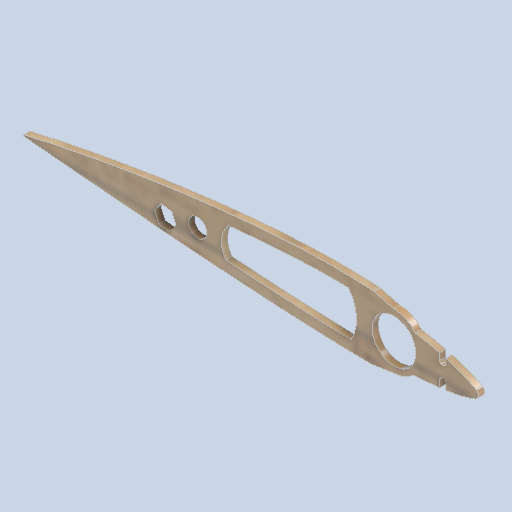
# Autodesk Inventor part: Rib V6 Flap BB
Saved by Autodesk Inventor 2025.2 (Build 292293000, 293)
## iProperties
Created: 2024-10-23
Part Number: Rib V6 Flap BB
Material: Wood (Maple)
Document SubType Name: Modeling
Designer: 17jo6
Density: 0.67 g/cm^3
Appearance: Natural Maple - Glossy Dark Tint
Author: 17jo6
Autodesk Inventor part; units mm, degrees
ref_plane "YZ Plane" through (0, 0, 0) normal (1, 0, 0) x (0, 1, 0)
ref_plane "XZ Plane" through (0, 0, 0) normal (0, 1, 0) x (-1, 0, 0)
ref_plane "XY Plane" through (0, 0, 0) normal (0, 0, 1) x (1, 0, 0)
sketch "Sketch1" plane through (0, 0, 0) normal (0, 0, 1) x (1, 0, 0)
  spline S0 degree 4 poles (254.436054, 38.258138) (252.159915, 38.650332) (246.788709, 39.499265) (237.984874, 40.618279) (225.357478, 41.704285) (211.202741, 42.341661) (196.392584, 42.47009) (181.031283, 42.070233) (165.506388, 41.221743) (149.785249, 40.04478) (134.1096, 38.577548) (118.624688, 36.850842) (103.500036, 34.939301) (88.901638, 32.883406) (74.995754, 30.738214) (61.917783, 28.562704) (49.827113, 26.40977) (38.835364, 24.340018) (29.07721, 22.403865) (20.632296, 20.65644) (13.645605, 19.149082) (6.913163, 17.660714) (2.90218, 16.740022) (0.469137, 16.188187) (0, 16.065) knots 0.21429705 0.21429705 0.21429705 0.21429705 0.21429705 0.2433201 0.28177524 0.32154178 0.36237973 0.40400459 0.44617789 0.48866482 0.5312306 0.57368816 0.61580317 0.65733642 0.6980466 0.73768213 0.77598623 0.81268845 0.84749504 0.88008735 0.91009265 0.93705903 0.9603631 1 1 1 1 1
  spline S1 degree 4 poles (299.999998, 15.624) (299.805651, 13.312974) (297.70854, 10.343184) (293.050897, 7.5008) (285.395888, 4.883043) (278.112378, 3.216454) (269.51472, 1.892454) (259.681019, 0.912997) (248.712883, 0.278332) (236.711867, -0.030891) (223.806667, -0.050368) (210.125319, 0.193333) (195.775416, 0.645033) (180.96771, 1.249367) (165.65166, 1.982539) (150.191633, 2.90484) (134.687258, 3.945111) (119.337536, 5.049498) (104.304232, 6.19869) (89.75661, 7.356132) (75.849241, 8.488651) (62.742943, 9.582403) (50.581067, 10.622604) (39.497088, 11.57965) (29.629376, 12.451281) (21.071247, 13.226368) (13.963939, 13.872105) (7.103576, 14.512622) (2.968279, 14.899676) (0.533018, 15.1397) (-0.004161, 15.184114) knots 0 0 0 0 0 0.05437224 0.07982113 0.10791215 0.1384988 0.1713415 0.2061871 0.24278378 0.28089063 0.3202767 0.36071301 0.4020228 0.44398485 0.4863729 0.52895769 0.5714601 0.61364209 0.65526508 0.6960853 0.73585299 0.77430798 0.81117416 0.84615676 0.87892978 0.90911464 0.93625212 0.9597112 1 1 1 1 1
  arc A0 (0, 16.065) -> (-0.004161, 15.184114) centre (0.115799, 15.624) ccw
  line L0 (0.115799, 15.624) -> (227.990221, 15.624) construction
  line L1 (299.999998, 15.624) -> (0.115799, 15.624) construction
  line L2 (299.999998, 15.624) -> (199.999998, 15.624) construction
  line L3 (199.999998, 15.624) -> (199.999998, 42.37734) construction
  line L4 (199.999998, 15.624) -> (199.999998, 0.52729)
  line L5 (0, 0) -> (0, 20.241)
  line L6 (0, 20.241) -> (238.581, 20.241) construction
  circle A1 centre (238.581, 20.241) radius 14
  line L7 (238.581, 20.241) -> (208.581, 20.241)
  line L8 (238.581, 25.359) -> (238.581, 20.241)
  line L9 (0, 20.241) -> (112, 20.241) construction
  circle A2 centre (112, 20.241) radius 5.39
  line L10 (0, 15.624) -> (112, 15.624) construction
  line L11 (0, 15.624) -> (112, 15.624) construction
  line L12 (112, 15.624) -> (112, 35.994456)
  line L13 (112, 15.624) -> (112, 5.61525)
  spline S2 degree 4 poles (299.285198, 20.241) (299.227939, 20.131643) (299.16804, 20.023225) (299.105573, 19.915754) (299.040612, 19.809235) knots 0 0 0 0 0 1 1 1 1 1
  line L14 (299.207055, 20.082158) -> (298.87417, 19.536312) construction
  arc A3 (298.903999, 19.593162) -> (299.170168, 20.029611) centre (292.291091, 23.925437) ccw construction
  line L15 (299.43203, 20.521431) -> (299.138367, 19.960569) construction
  arc A4 (299.163926, 20.01882) -> (299.398715, 20.467241) centre (292.801001, 23.636075) ccw construction
  spline S3 degree 2 poles (295.850621, 16.559978) (295.157262, 16.069203) (294.393311, 15.624) knots 0 0 0 1 1 1
  line L16 (294.550692, 15.715716) -> (294.235931, 15.532284) construction
  arc A5 (294.267154, 15.551069) -> (294.518956, 15.69781) centre (283.884356, 33.65696) ccw construction
  spline S4 degree 4 poles (296.856901, 15.624) (296.618326, 15.862944) (296.370731, 16.098547) (296.114674, 16.330852) (295.850621, 16.559978) knots 0 0 0 0 0 1 1 1 1 1
  spline S5 degree 4 poles (219.58717, 34.91187) (218.695351, 34.95198) (214.858509, 35.106335) (210.707211, 35.329502) (192.898023, 35.446366) (181.42777, 35.055508) (165.177387, 34.181901) (149.561876, 33.12667) (133.828431, 31.347909) (128.265438, 31.097419) (123.390775, 30.590026) knots 0 0 0 0 0 0.13924435 0.23321956 0.36393672 0.50998276 0.65711487 0.7981047 1 1 1 1 1
  line L17 (295.959293, 16.465681) -> (295.74195, 16.654276) construction
  arc A6 (295.937354, 16.484307) -> (295.763482, 16.635181) centre (281.87292, 0.451609) ccw construction
  line L18 (232.743774, 34.364452) -> (201.193566, 35.681454) construction
  arc A7 (229.586762, 34.454933) -> (204.347135, 35.508511) centre (136.348344, -1896.324468) ccw construction
  arc A8 (264.266057, 15.123) -> (264.360826, 15.624) centre (238.581, 20.241) ccw
  circle A9 centre (238.581, 20.241) radius 24
  circle A10 centre (112, 20.241) radius 15.39
  spline S6 degree 4 poles (299.999998, 15.624) (300.269142, 17.933652) (298.783415, 21.267693) (294.693448, 24.979847) (287.53174, 28.940551) (280.486947, 31.820538) (271.480983, 34.718213) (262.486804, 36.793013) (257.700386, 37.695672) (254.436054, 38.258138) knots 0 0 0 0 0 0.24755477 0.36385739 0.4925498 0.63299607 0.77826439 1 1 1 1 1
  line L19 (285.294543, 32.941011) -> (223.577565, 43.575266) construction
  arc A11 (278.722442, 32.634865) -> (229.668212, 41.087243) centre (217.218351, -177.738587) ccw construction
  line L20 (285.294543, 32.941011) -> (223.577565, 43.575266) construction
  arc A12 (278.877125, 33.041766) -> (229.658629, 41.522447) centre (200.894914, -272.473312) ccw construction
  spline S7 degree 4 poles (251.493, 31.73616) (243.700929, 32.967588) (232.160237, 34.296592) (216.442824, 35.287928) (196.392341, 35.461091) (181.031705, 35.061513) (165.505292, 34.212684) (149.788285, 33.036509) (134.101234, 31.567156) (118.647366, 29.846206) (103.439709, 27.919279) (89.058912, 25.903716) (74.837064, 23.692714) (62.488433, 21.669546) (49.639937, 19.354465) (46.379459, 18.742869) (43.812536, 18.259032) knots 0 0 0 0 0 0.1639631 0.23233838 0.3020312 0.37264227 0.44377843 0.51504665 0.58613365 0.65664712 0.72618654 0.7943479 0.86070997 0.92034602 1 1 1 1 1
  spline S8 degree 4 poles (295.845009, 16.556007) (295.719822, 16.664559) (294.584958, 17.628339) (292.058546, 19.428263) (287.516704, 21.93465) (280.467029, 24.832118) (271.97142, 27.522599) (264.208658, 29.400369) (258.409244, 30.551465) (255.053616, 31.142888) (254.436054, 31.249298) (253.968946, 31.329784) (253.501839, 31.41027) (253.034731, 31.490756) (252.567623, 31.571241) knots 0 0 0 0 0 0.01890503 0.16895946 0.33499927 0.51620401 0.71116085 0.9183366 0.96483207 0.96483207 0.96483207 0.96483207 1 1 1 1 1
  line L21 (285.294543, 25.932171) -> (223.577565, 36.566425) construction
  line L22 (285.294543, 25.932171) -> (223.577565, 36.566425) construction
  arc A13 (278.722442, 25.626025) -> (229.668212, 34.078402) centre (217.218351, -184.747428) ccw construction
  line L23 (270.129, 9.125374) -> (275.129, 9.125374) construction
  line L24 (281.07, 24.45816) -> (286.07, 24.45816) construction
  line L25 (318.821413, -3.367269) -> (272.868604, 36.479282) construction
  arc A14 (303.207925, 0.551953) -> (278.959518, 21.578206) centre (281.857648, 0.425162) ccw construction
  spline S9 degree 4 poles (295.835285, 16.564433) (293.417091, 14.88464) (288.41352, 12.692641) (280.70627, 10.669821) (269.511023, 8.939829) (259.682627, 7.96324) (248.712204, 7.32734) (236.712148, 7.018633) (223.806545, 6.998947) (210.125394, 7.242728) (195.775305, 7.694406) (180.967993, 8.298721) (165.65086, 9.03198) (150.193891, 9.954022) (134.681006, 10.995018) (119.354518, 12.097424) (104.258979, 13.251926) (89.874814, 14.39542) (75.752353, 15.547068) (62.906491, 16.616479) (50.510696, 17.677636) (46.516568, 18.024605) (43.812536, 18.259032) knots 0 0 0 0 0 0.08476672 0.12402522 0.16617938 0.21090431 0.25787677 0.30678758 0.35734028 0.40924097 0.46226281 0.51612182 0.5705276 0.62518592 0.67973848 0.7338798 0.78730362 0.83969707 0.89073959 0.93714265 1 1 1 1 1
  spline S10 degree 4 poles (21.462276, 20.241) (20.622656, 20.316984) (20.124028, 20.362207) (19.919133, 20.380856) (19.554048, 20.414029) knots 0 0 0 0 0 1 1 1 1 1 construction
  line L26 (68.488377, 16.119755) -> (19.136695, 20.398308) construction
  arc A15 (63.551474, 16.528056) -> (24.070206, 19.950891) centre (-819.899413, -9944.371227) ccw construction
  line L27 (21.724437, 20.217275) -> (21.200116, 20.264725) construction
  arc A16 (21.252548, 20.259982) -> (21.672005, 20.222022) centre (898.635849, 9712.955601) ccw construction
  line L28 (74.254065, 23.996937) -> (13.371006, 12.521126) construction
  arc A17 (68.175943, 22.793945) -> (19.469999, 13.613391) centre (1053.390082, -5337.891027) ccw construction
  spline S11 degree 4 poles (218.437499, 7.193419) (217.617295, 7.240848) (213.819214, 7.468804) (209.586315, 6.850678) (192.548492, 7.944114) (181.146901, 8.16297) (165.746092, 9.02826) (149.142366, 9.880106) (139.977668, 10.751942) (129.107316, 11.246393) (124.68665, 11.528881) knots 0 0 0 0 0 0.12763083 0.21372336 0.33362841 0.4674456 0.60262129 0.73842442 0.88039529 0.88039529 0.88039529 0.88039529 0.88039529
  line L29 (133.533683, 10.96354) -> (115.839617, 12.094223) construction
  arc A18 (117.617989, 12.078874) -> (131.767822, 11.174674) centre (141.026952, 267.238396) ccw construction
  line L30 (140.664975, 32.388062) -> (106.116576, 28.79199) construction
  arc A19 (137.221962, 31.449676) -> (109.679039, 28.58279) centre (140.622493, -134.959578) ccw construction
  circle A20 centre (238.581, 20.241) radius 18
  line L31 (238.581, 38.241) -> (225.78, 41.559)
  line L32 (238.581, 2.241) -> (224.22, 0)
  line L33 (214.581, 20.241) -> (214.581, 42.126574) construction
  line L34 (127.39, 20.241) -> (127.39, 11.525517) construction
  line L35 (127.39, 20.241) -> (131.31394, 20.241) construction
  line L36 (96.61, 20.241) -> (96.61, 13.863077) construction
  line L37 (270.129, 5.61525) -> (270.129, 15.624) construction
  line L38 (272.129, 7.61525) -> (272.129, 13.624)
  line L39 (268.129, 13.624) -> (268.129, 7.61525)
  arc A21 (268.129, 7.61525) -> (272.129, 7.61525) centre (270.129, 7.61525) ccw
  arc A22 (272.129, 13.624) -> (268.129, 13.624) centre (270.129, 13.624) ccw
  line L40 (270.129, 32.18075) -> (270.129, 22.172) construction
  line L41 (272.129, 30.18075) -> (272.129, 24.172)
  line L42 (268.129, 24.172) -> (268.129, 30.18075)
  arc A23 (272.129, 30.18075) -> (268.129, 30.18075) centre (270.129, 30.18075) ccw
  arc A24 (268.129, 24.172) -> (272.129, 24.172) centre (270.129, 24.172) ccw
  arc A25 (199.999998, 42.31547) -> (199.853854, 42.377258) centre (190.581, 20.241) ccw
  arc A26 (171.272979, 34.495835) -> (171.268099, 34.489223) centre (190.581, 20.241) ccw
  arc A27 (210.748391, 7.230376) -> (209.287499, 35.276521) centre (190.581, 20.241) ccw
  arc A28 (169.44554, 8.870309) -> (169.474435, 8.816763) centre (190.581, 20.241) ccw
  arc A29 (153.976817, 9.682431) -> (154.030254, 9.739387) centre (142.78, 20.241) ccw
  arc A30 (151.241916, 33.095886) -> (151.219343, 33.110716) centre (142.78, 20.241) ccw
  arc A31 (132.12991, 31.350801) -> (130.322928, 11.203663) centre (142.78, 20.241) ccw
  arc A32 (95.274104, 13.969298) -> (95.169771, 26.74146) centre (81.22, 20.241) ccw
  arc A33 (66.333989, 16.334751) -> (66.538876, 15.624) centre (81.22, 20.241) ccw
  line L43 (112, 20.241) -> (112, 14.851) construction
  circle A34 centre (91.265, 15.422) radius 4
  circle A35 centre (238.581, 20.241) radius 14.2
  circle A36 centre (112, 20.241) radius 5.92
  circle A37 centre (91.265, 15.422) radius 6
  line L44 (98.144895, 14.605275) -> (93.997643, 9.055474)
  line L45 (93.997643, 9.055474) -> (87.117748, 9.872198)
  line L46 (87.117748, 9.872198) -> (84.385105, 16.238725)
  line L47 (84.385105, 16.238725) -> (88.532357, 21.788526)
  line L48 (88.532357, 21.788526) -> (95.412252, 20.971802)
  line L49 (95.412252, 20.971802) -> (98.144895, 14.605275)
  point P0 (0.783, 16.254)
  point P1 (3.213, 16.812)
  point P2 (7.239, 17.724)
  point P3 (12.813, 18.96)
  point P4 (19.884, 20.484)
  point P5 (28.374, 22.245)
  point P6 (38.199, 24.195)
  point P7 (49.254, 26.28)
  point P8 (61.419, 28.446)
  point P9 (74.571, 30.636)
  point P10 (88.56, 32.793)
  point P11 (103.242, 34.86)
  point P12 (118.455, 36.783)
  point P13 (134.028, 38.511)
  point P14 (149.793, 39.984)
  point P15 (165.576, 41.16)
  point P16 (181.206, 41.985)
  point P17 (196.638, 42.363)
  point P18 (211.554, 42.222)
  point P19 (239.145, 40.389)
  point P20 (262.68, 36.666)
  point P21 (272.577, 34.218)
  point P22 (281.07, 31.467)
  point P23 (288.069, 28.491)
  point P24 (293.505, 25.359)
  point P25 (297.324, 22.137)
  point P26 (300, 15.624)
  point P27 (0.861, 15.105)
  point P28 (3.342, 14.868)
  point P29 (7.446, 14.481)
  point P30 (13.122, 13.953)
  point P31 (20.31, 13.296)
  point P32 (28.92, 12.519)
  point P33 (38.856, 11.64)
  point P34 (50.007, 10.674)
  point P35 (62.244, 9.63)
  point P36 (75.429, 8.529)
  point P37 (89.418, 7.389)
  point P38 (104.052, 6.228)
  point P39 (119.172, 5.076)
  point P40 (134.613, 3.966)
  point P41 (150.207, 2.928)
  point P42 (165.783, 2.013)
  point P43 (181.167, 1.263)
  point P44 (196.068, 0.663)
  point P45 (210.468, 0.225)
  point P46 (237.189, 0.039)
  point P47 (249.246, 0.378)
  point P48 (260.262, 1.05)
  point P49 (270.129, 2.076)
  point P50 (278.739, 3.462)
  point P51 (285.993, 5.211)
  point P52 (291.81, 7.314)
  point P53 (296.121, 9.756)
  point P54 (298.863, 12.531)
  point P55 (199.999998, 15.624)
  point P56 (225.364219, 15.624)
  point P57 (238.581, 6.241)
  point P58 (238.581, 34.241)
  point P59 (225.364219, 15.624)
  point P60 (251.797781, 15.624)
  point P61 (0, 16.065)
  point P62 (0, 15.183769)
  point P63 (224.581, 20.241)
  point P64 (112, 25.631)
  point P65 (0, 9.065)
  point P66 (0.783, 9.254)
  point P67 (3.213, 9.812)
  point P68 (7.239, 10.724)
  point P69 (12.813, 11.96)
  point P70 (19.884, 13.484)
  point P71 (28.374, 15.245)
  point P72 (38.199, 17.195)
  point P73 (49.254, 19.28)
  point P74 (61.419, 21.446)
  point P75 (74.571, 23.636)
  point P76 (88.56, 25.793)
  point P77 (103.242, 27.86)
  point P78 (118.455, 29.783)
  point P79 (134.028, 31.511)
  point P80 (149.793, 32.984)
  point P81 (165.576, 34.16)
  point P82 (181.206, 34.985)
  point P83 (225.78, 34.559)
  point P84 (239.145, 33.389)
  point P85 (251.493, 31.745)
  point P86 (262.68, 29.666)
  point P87 (272.577, 27.218)
  point P88 (281.07, 24.467)
  point P89 (288.069, 21.491)
  point P90 (293.505, 18.359)
  point P91 (297.324, 15.137)
  point P92 (299.493, 11.879)
  point P93 (300, 8.624)
  point P94 (-0.004161, 22.184114)
  point P95 (0.861, 22.105)
  point P96 (3.342, 21.868)
  point P97 (7.446, 21.481)
  point P98 (13.122, 20.953)
  point P99 (20.31, 20.296)
  point P100 (28.92, 19.519)
  point P101 (38.856, 18.64)
  point P102 (50.007, 17.674)
  point P103 (62.244, 16.63)
  point P104 (75.429, 15.529)
  point P105 (89.418, 14.389)
  point P106 (104.052, 13.228)
  point P107 (119.172, 12.076)
  point P108 (134.613, 10.966)
  point P109 (150.207, 9.928)
  point P110 (165.783, 9.013)
  point P111 (181.167, 8.263)
  point P112 (196.068, 7.663)
  point P113 (210.468, 7.225)
  point P114 (224.22, 7)
  point P115 (237.189, 7.039)
  point P116 (249.246, 7.378)
  point P117 (260.262, 8.05)
  point P118 (270.129, 9.076)
  point P119 (278.739, 10.462)
  point P120 (285.993, 12.211)
  point P121 (291.81, 14.314)
  point P122 (296.121, 16.756)
  point P123 (298.863, 19.531)
  point P124 (300, 22.624)
  point P125 (18.740477, 20.241)
  point P126 (216.96867, 35.022953)
  point P127 (0, 16.065)
  point P128 (296.856901, 15.624)
  point P129 (294.393311, 15.624)
  point P130 (219.58717, 34.91187)
  point P131 (123.390775, 30.590026)
  point P132 (254.436054, 38.258138)
  point P133 (0, 9.05616)
  point P134 (0.783, 9.24516)
  point P135 (3.213, 9.80316)
  point P136 (7.239, 10.71516)
  point P137 (12.813, 11.95116)
  point P138 (19.884, 13.47516)
  point P139 (28.374, 15.23616)
  point P140 (38.199, 17.18616)
  point P141 (49.254, 19.27116)
  point P142 (61.419, 21.43716)
  point P143 (74.571, 23.62716)
  point P144 (88.56, 25.78416)
  point P145 (103.242, 27.85116)
  point P146 (118.455, 29.77416)
  point P147 (134.028, 31.50216)
  point P148 (149.793, 32.97516)
  point P149 (165.576, 34.15116)
  point P150 (181.206, 34.97616)
  point P151 (196.638, 35.35416)
  point P152 (211.554, 35.21316)
  point P153 (225.78, 34.55016)
  point P154 (262.68, 29.65716)
  point P155 (272.577, 27.20916)
  point P156 (297.324, 15.12816)
  point P157 (299.493, 11.87016)
  point P158 (300, 8.61516)
  point P159 (254.436054, 31.249298)
  point P160 (216.884838, -206.362485)
  point P161 (278.876889, 26.073396)
  point P162 (229.590604, 33.866167)
  point P163 (-0.004161, 22.233488)
  point P164 (0.861, 22.154374)
  point P165 (3.342, 21.917374)
  point P166 (7.446, 21.530374)
  point P167 (13.122, 21.002374)
  point P168 (28.92, 19.568374)
  point P169 (38.856, 18.689374)
  point P170 (50.007, 17.723374)
  point P171 (62.244, 16.679374)
  point P172 (75.429, 15.578374)
  point P173 (89.418, 14.438374)
  point P174 (104.052, 13.277374)
  point P175 (119.172, 12.125374)
  point P176 (134.613, 11.015374)
  point P177 (150.207, 9.977374)
  point P178 (165.783, 9.062374)
  point P179 (181.167, 8.312374)
  point P180 (196.068, 7.712374)
  point P181 (210.468, 7.274374)
  point P182 (224.22, 7.049374)
  point P183 (237.189, 7.088374)
  point P184 (249.246, 7.427374)
  point P185 (260.262, 8.099374)
  point P186 (278.739, 10.511374)
  point P187 (285.993, 12.260374)
  point P188 (296.121, 16.805374)
  point P189 (298.863, 19.580374)
  point P190 (300, 22.673374)
  point P191 (225.700031, -0.009448)
  point P192 (252.261653, 0.521981)
  point P193 (227.349521, 41.450759)
  point P194 (105.977751, 6.07821)
  point P195 (115.800844, 5.327728)
  point P196 (98.259993, 27.173842)
  point P197 (260.452219, 30.122789)
  point P198 (123.585295, 30.371797)
  point P199 (134.59788, 31.560388)
  dimension "d38" = 10.78
  dimension "d68" = 12
  dimension "d17" = 100
  dimension "d19" = 20.241
  dimension "d20" = 238.581
  dimension "d21" = 28
  dimension "d37" = 112
  dimension "d39" = 112
  dimension "d40" = 0
  dimension "d43" = 10
  dimension "d44" = 10
  dimension "d55" = 4
  dimension "d56" = 90
  dimension "d58" = 4
  dimension "d60" = 8
  dimension "d63" = 20.735
  dimension "d66" = 28.4
  dimension "d67" = 11.84
  constraints: 103 end point, 61 point on circle, 36 centre point, 31 midpoint, 21 point on line, 7 horizontal, 7 tangent, 6 coincident, 6 perpendicular, 3 collinear, 3 symmetric about line, 1 horizontal alignment, 1 parallel, 1 vertical, 208 other
  measures "d17" distance of L1.start L2.end
  measures "d19" distance of L5.start L5.end
  measures "d20" distance of L5.end L6.end
  measures "d21" diameter of A1
  measures "d37" distance of L5.end L9.end
  measures "d39" distance of L10.start L10.end
  measures "d40" distance between parallel lines of L11 L10
  measures "d43" radial gap between concentric circles of A1 A9
  measures "d55" radial gap between concentric circles of A1 A20
  measures "d56" angle of L34 L35
  measures "d58" diameter of A22
  measures "d60" diameter of A34
  measures "d63" distance from line of L13 A34.centre
  measures "d66" diameter of A35
  measures "d67" diameter of A36
sketch "Sketch1 outline for Extrusion3" plane through (0, 0, 0) normal (0, 0, 1) x (1, 0, 0)
  arc A0 (130.322928, 11.203663) -> (132.12991, 31.350801) centre (142.78, 20.241) cw
  spline S0 degree 4 poles (134.59788, 31.560388) (133.959991, 31.50476) (133.336858, 31.451452) (132.727643, 31.400296) (132.12991, 31.350801) knots 0 0 0 0 0 1 1 1 1 1
  spline S1 degree 4 poles (148.35454, 32.852821) (146.744748, 32.714531) (143.299889, 32.409801) (139.858916, 32.086834) (136.425249, 31.746516) (134.59788, 31.560388) knots 0 0 0 0 0 0.46716356 1 1 1 1 1
  spline S2 degree 4 poles (168.289351, 34.321059) (165.616538, 34.166288) (160.663613, 33.861392) (155.902937, 33.52597) (150.772624, 33.075904) (148.35454, 32.852821) knots 0 0 0 0 0 0.53453464 1 1 1 1 1
  spline S3 degree 4 poles (178.528633, 34.863187) (177.234649, 34.805508) (174.676887, 34.68378) (172.117601, 34.547428) (169.555533, 34.397953) (168.289351, 34.321059) knots 0 0 0 0 0 0.50607706 1 1 1 1 1
  spline S4 degree 4 poles (200.033241, 35.36854) (196.989538, 35.373098) (190.993259, 35.339534) (186.178785, 35.202371) (181.085446, 34.98454) (178.528633, 34.863187) knots 0 0 0 0 0 0.51135579 1 1 1 1 1
  spline S5 degree 4 poles (205.775807, 35.331387) (205.328945, 35.337353) (203.897941, 35.354391) (202.462975, 35.36488) (201.024133, 35.368857) (200.033241, 35.36854) knots 0 0 0 0 0 0.31254487 1 1 1 1 1
  spline S6 degree 4 poles (209.287499, 35.276521) (208.497769, 35.292495) (207.648728, 35.30713) (206.737448, 35.320194) (205.775807, 35.331387) knots 0 0 0 0 0 1 1 1 1 1
  arc A1 (209.287499, 35.276521) -> (209.293312, 35.269287) centre (190.581, 20.241) cw
  arc A2 (209.293312, 35.269287) -> (210.772015, 7.267069) centre (190.581, 20.241) cw
  spline S7 degree 4 poles (211.556221, 7.248653) (211.360299, 7.253176) (211.164291, 7.257753) (210.968196, 7.262384) (210.772015, 7.267069) knots 0 0 0 0 0 1 1 1 1 1
  spline S8 degree 4 poles (211.556221, 7.248653) (211.431947, 7.24563) (209.712471, 7.204499) (205.181462, 7.133368) (192.548492, 7.944114) (181.146901, 8.16297) (165.746092, 9.02826) (150.424265, 9.814339) (141.886646, 10.576084) (133.759076, 11.015279) (130.322928, 11.203663) knots 0 0 0 0 0 0.00945218 0.12946997 0.29662431 0.48317293 0.6716154 0.86093254 1 1 1 1 1
  spline S9 degree 4 poles (224.22, 0) (222.479951, 0.013004) (217.292297, 0.069187) (208.469243, 0.245463) (195.775416, 0.645033) (180.96771, 1.249367) (165.65166, 1.982539) (150.191633, 2.90484) (134.687258, 3.945111) (119.337536, 5.049498) (104.304232, 6.19869) (89.75661, 7.356132) (75.849241, 8.488651) (62.742943, 9.582403) (50.581067, 10.622604) (39.497088, 11.57965) (29.629376, 12.451281) (21.071247, 13.226368) (13.963939, 13.872105) (7.107973, 14.512211) (2.97534, 14.899015) (0.541913, 15.138823) (0, 15.183769) knots 0 0 0 0 0 0.02936819 0.08711706 0.14611338 0.20604122 0.26657745 0.32739466 0.3880942 0.44833615 0.50777977 0.56607692 0.6228709 0.67779016 0.73044036 0.78040055 0.82720513 0.87031346 0.90906968 0.94257262 1 1 1 1 1
  line L0 (224.22, 0) -> (238.581, 2.241)
  arc A3 (238.581, 2.241) -> (251.319332, 7.523497) centre (238.581, 20.241) ccw
  spline S10 degree 4 poles (268.129, 8.876482) (267.350973, 8.784165) (264.070152, 8.41388) (259.922783, 8.03946) (255.648904, 7.749196) (252.134203, 7.563785) (251.319332, 7.523497) knots 0 0 0 0 0 0.19446677 0.81409157 1 1 1 1 1
  line L1 (268.129, 8.876482) -> (268.129, 13.624)
  arc A4 (268.129, 13.624) -> (272.129, 13.624) centre (270.129, 13.624) cw
  line L2 (272.129, 13.624) -> (272.129, 9.39886)
  spline S11 degree 4 poles (295.835285, 16.564433) (293.417091, 14.88464) (288.41352, 12.692641) (282.206639, 11.063603) (275.277329, 9.862415) (272.65595, 9.474358) (272.129, 9.39886) knots 0 0 0 0 0 0.63339451 0.92674211 1 1 1 1 1
  spline S12 degree 4 poles (295.835285, 16.564433) (295.712426, 16.670837) (294.579422, 17.632282) (292.055318, 19.430045) (287.516704, 21.93465) (281.462074, 24.423147) (276.515305, 26.06668) (273.276333, 27.014249) (272.129, 27.335374) knots 0 0 0 0 0 0.03023743 0.27499105 0.54581841 0.84138126 1 1 1 1 1
  line L3 (272.129, 27.335374) -> (272.129, 24.172)
  arc A5 (272.129, 24.172) -> (268.129, 24.172) centre (270.129, 24.172) cw
  line L4 (268.129, 24.172) -> (268.129, 28.393044)
  spline S13 degree 4 poles (268.129, 28.393044) (267.95313, 28.436967) (265.243797, 29.109201) (261.874729, 29.863619) (258.409244, 30.551465) (255.053616, 31.142888) (254.436054, 31.249298) (253.968946, 31.329784) (253.501839, 31.41027) (253.034731, 31.490756) (252.567623, 31.571241) knots 0 0 0 0 0 0.04751866 0.73070527 0.88402957 0.88402957 0.88402957 0.88402957 1 1 1 1 1
  arc A6 (252.567623, 31.571241) -> (238.581, 38.241) centre (238.581, 20.241) ccw
  line L5 (238.581, 38.241) -> (225.78, 41.559)
  spline S14 degree 4 poles (225.78, 41.559) (223.981701, 41.678798) (218.618296, 41.998081) (209.491978, 42.356496) (196.392584, 42.47009) (181.031283, 42.070233) (165.506388, 41.221743) (149.785249, 40.04478) (134.1096, 38.577548) (118.624688, 36.850842) (103.500036, 34.939301) (88.901638, 32.883406) (74.995754, 30.738214) (61.917783, 28.562704) (49.827113, 26.40977) (38.835364, 24.340018) (29.07721, 22.403865) (20.632296, 20.65644) (13.645605, 19.149082) (6.913163, 17.660714) (2.90218, 16.740022) (0.469137, 16.188187) (0, 16.065) knots 0 0 0 0 0 0.02971241 0.08811623 0.14764545 0.20795901 0.26872109 0.32959596 0.39031605 0.45054625 0.50994444 0.56816554 0.62484975 0.67962982 0.73211898 0.78189715 0.82850859 0.87142025 0.90998584 0.94331385 1 1 1 1 1
  arc A7 (0, 16.065) -> (-0.004161, 15.184114) centre (0.115799, 15.624) ccw
  spline S15 degree 4 poles (0, 15.183769) (-0.001046, 15.183856) (-0.002088, 15.183942) (-0.003126, 15.184028) (-0.004161, 15.184114) knots 0 0 0 0 0 1 1 1 1 1
  line L6 (95.412252, 20.971802) -> (98.144895, 14.605275)
  line L7 (98.144895, 14.605275) -> (93.997643, 9.055474)
  line L8 (93.997643, 9.055474) -> (87.117748, 9.872198)
  line L9 (87.117748, 9.872198) -> (84.385105, 16.238725)
  line L10 (84.385105, 16.238725) -> (88.532357, 21.788526)
  line L11 (88.532357, 21.788526) -> (95.412252, 20.971802)
  circle A8 centre (112, 20.241) radius 5.92
  spline S16 degree 4 poles (244.30613, 7.246275) (244.166974, 7.242058) (244.027727, 7.237902) (243.88839, 7.233805) (243.748965, 7.229769) knots 0 0 0 0 0 1 1 1 1 1
  arc A9 (243.748965, 7.229769) -> (245.021033, 32.671848) centre (238.581, 20.241) cw
  spline S17 degree 4 poles (245.576846, 32.598109) (245.438039, 32.616675) (245.299134, 32.635153) (245.160132, 32.653544) (245.021033, 32.671848) knots 0 0 0 0 0 1 1 1 1 1
  arc A10 (245.576846, 32.598109) -> (244.30613, 7.246275) centre (238.581, 20.241) cw
extrude "Extrusion3" add sketch "Sketch1 outline for Extrusion3" along normal blind 4
fillet "Fillet4" radius 3 1 edges at (295.8353, 16.5644, 2)
body "Solid2"
